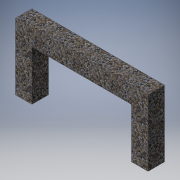
# Autodesk Inventor part: RailsMini
Saved by Autodesk Inventor 2016 (Build 200138000, 138)
## iProperties
Created: 2015-08-15
Part Number: RailsMini
Material: Concrete
Document SubType Name: Modeling
Designer: myhome
Density: 2.40731 g/cm^3
Appearance: Exposed Aggregate - Coarse
Mass: 33702.4 g
Surface Area: 5800 cm^2
Volume: 14000 cm^3
Author: myhome
Autodesk Inventor part; units mm, degrees
ref_plane "YZ Plane" through (0, 0, 0) normal (1, 0, 0) x (0, 1, 0)
ref_plane "XZ Plane" through (0, 0, 0) normal (0, 1, 0) x (-1, 0, 0)
ref_plane "XY Plane" through (0, 0, 0) normal (0, 0, 1) x (1, 0, 0)
sketch "Sketch1" plane through (0, 0, 0) normal (0, 0, 1) x (1, 0, 0)
  line L0 (0, 0) -> (0, 400)
  line L1 (0, 400) -> (800, 400)
  line L2 (800, 400) -> (800, 0)
  line L3 (800, 0) -> (700, 0)
  line L4 (700, 0) -> (700, 300)
  line L5 (700, 300) -> (100, 300)
  line L6 (100, 300) -> (100, 0)
  line L7 (100, 0) -> (0, 0)
  dimension "d0" = 400
  dimension "d1" = 800
  dimension "d2" = 400
  dimension "d3" = 100
  dimension "d4" = 300
  dimension "d5" = 600
  dimension "d6" = 300
  dimension "d7" = 100
  constraints: 16 end point, 5 perpendicular, 1 point on line, 1 vertical
  measures "d0" distance of L0.start L0.end
  measures "d1" distance of L0.end L1.end
  measures "d2" distance of L1.end L2.end
  measures "d3" distance of L2.end L3.end
  measures "d4" distance of L3.end L4.end
  measures "d5" distance of L4.end L5.end
  measures "d6" distance of L5.end L6.end
  measures "d7" distance of L6.end L0.start
extrude "Extrusion1" add sketch "Sketch1" against normal blind 100
body "Solid1"
